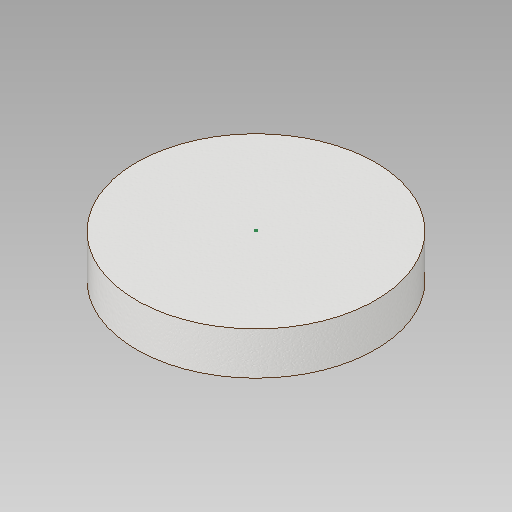
# Autodesk Inventor part: 使用タイヤ　スポンジ部分
Saved by Autodesk Inventor 2017 (Build 210142000, 142)
## iProperties
Part Number: 使用タイヤ　スポンジ部分
Material: ポリウレタン フォーム
Document SubType Name: Modeling
Designer: HISAAKI
Density: 0.032 g/cm^3
Appearance: 粗い テクスチャ - 暗褐色
Mass: 12.0009 g
Surface Area: 425.686 cm^2
Volume: 375.028 cm^3
Author: HISAAKI
Autodesk Inventor part; units mm, degrees
ref_plane "YZ Plane" through (0, 0, 0) normal (1, 0, 0) x (0, 1, 0)
ref_plane "XZ Plane" through (0, 0, 0) normal (0, 1, 0) x (-1, 0, 0)
ref_plane "XY Plane" through (0, 0, 0) normal (0, 0, 1) x (1, 0, 0)
sketch "スケッチ1" plane through (0, 0, 0) normal (0, 1, 0) x (-1, 0, 0)
  circle A0 centre (0, 0) radius 70
  dimension "d0" = 140
  constraints: 1 centre point, 1 coincident
  measures "d0" diameter of A0
extrude "押し出し1" add sketch "スケッチ1" along normal blind 25
sketch "スケッチ2" plane through (0, 0, 0) normal (0, -1, 0) x (1, 0, 0)
  circle A0 centre (0, 0) radius 25
  dimension "d3" = 50
  constraints: 1 centre point, 1 coincident
  measures "d3" diameter of A0
extrude "押し出し2" cut sketch "スケッチ2" against normal blind 5
sketch "スケッチ3" plane through (0, 25, 0) normal (0, 1, 0) x (1, 0, 0)
  point P0 (0, 0)
